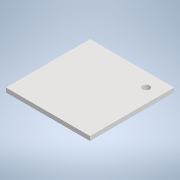
# Autodesk Inventor part: moving plate
Saved by Autodesk Inventor 2020 (Build 240168000, 168)
## iProperties
Created: 2021-02-27
Part Number: moving plate
Material: Generic
Document SubType Name: Modeling
Designer: Bernard Li
Density: 1 g/cm^3
Appearance: Default
Author: Bernard Li
Autodesk Inventor part; units mm, degrees
ref_plane "YZ Plane" through (0, 0, 0) normal (1, 0, 0) x (0, 1, 0)
ref_plane "XZ Plane" through (0, 0, 0) normal (0, 1, 0) x (-1, 0, 0)
ref_plane "XY Plane" through (0, 0, 0) normal (0, 0, 1) x (1, 0, 0)
sketch "Sketch1" plane through (0, 0, 0) normal (0, 1, 0) x (-1, 0, 0)
  line L0 (0, 0) -> (76.2, 0)
  line L1 (76.2, 0) -> (76.2, 76.2)
  line L2 (76.2, 76.2) -> (0, 76.2)
  line L3 (0, 76.2) -> (0, 0)
  dimension "d0" = 76.2
  dimension "d1" = 76.2
  constraints: 8 end point, 2 parallel, 1 horizontal, 1 perpendicular
  measures "d0" distance of L2.end L1.end
  measures "d1" distance of L1.end L0.end
extrude "Extrusion1" add sketch "Sketch1" along normal blind 3.81
sketch "Sketch2" plane through (0, 3.81, 0) normal (0, 1, 0) x (1, 0, 0)
  circle A0 centre (-12.7, -12.7) radius 12.7
  circle A1 centre (-12.7, -12.7) radius 3.175
  line L0 (0, 0) -> (-76.2, 0) projected
  line L1 (0, -76.2) -> (0, 0) projected
  dimension "d4" = 25.4
  constraints: 2 centre point, 2 tangent, 1 coincident
  measures "d4" diameter of A0
extrude "Extrusion2" cut sketch "Sketch2" against normal blind 3.81 contours A1
sketch "Sketch3" plane through (0, 0, 0) normal (0, -1, 0) x (1, 0, 0)
  circle A0 centre (-12.7, 12.7) radius 3.175 projected
  circle A1 centre (-12.7, 12.7) radius 12.7
  line L0 (0, 76.2) -> (0, 0) projected
  line L1 (0, 0) -> (-76.2, 0) projected
  line L2 (-12.7, 0) -> (0, 0)
  line L3 (0, 0) -> (0, 12.7)
  constraints: 4 end point, 2 point on circle, 2 point on line, 2 tangent, 1 centre point, 1 coincident, 1 collinear
extrude "Extrusion3" cut sketch "Sketch3" against normal blind 3.81 contours L0 L1 A1
fillet "Fillet1" radius 25.4 2 edges at (-76.2, 1.905, 76.2) (0, 1.905, 76.2)
body "Solid1"
